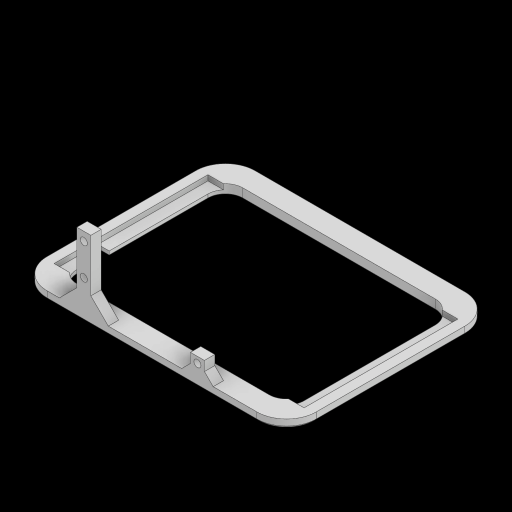
# Autodesk Inventor part: 220_Frame_Mainboard
Saved by Autodesk Inventor 2024 (Build 280153000, 153)
## iProperties
Created: 2023-07-20
Part Number: 220_Frame_Mainboard
Material: Generisch
Document SubType Name: Modeling
Designer: Philipp
Density: 1 g/cm^3
Appearance: Vorgabe
Author: Philipp
Autodesk Inventor part; units mm, degrees
ref_plane "YZ Plane" through (0, 0, 0) normal (1, 0, 0) x (0, 1, 0)
ref_plane "XZ Plane" through (0, 0, 0) normal (0, 1, 0) x (-1, 0, 0)
ref_plane "XY Plane" through (0, 0, 0) normal (0, 0, 1) x (1, 0, 0)
sketch "Skizze1" plane through (0, 0, 0) normal (0, 0, 1) x (1, 0, 0)
  line L0 (-77, 59.5) -> (77, 59.5)
  line L1 (77, 59.5) -> (77, -59.5)
  line L2 (77, -59.5) -> (-77, -59.5)
  line L3 (-77, -59.5) -> (-77, 59.5)
  line L4 (-77, 59.5) -> (77, -59.5) construction
  line L5 (77, 59.5) -> (-77, -59.5) construction
  point P0 (0, 0)
  dimension "d0" = 154
  dimension "d1" = 119
  constraints: 12 end point, 2 midpoint, 2 parallel, 1 horizontal, 1 perpendicular
  measures "d0" distance of L1.end L2.end
  measures "d1" distance of L0.end L1.end
extrude "Extrusion1" add sketch "Skizze1" along normal blind 5
fillet "Rundung1" radius 17 4 edges at (77, 59.5, 2.5) (77, -59.5, 2.5) (-77, -59.5, 2.5) (-77, 59.5, 2.5)
chamfer "Fasen1" distance 1.5 angle 45 8 edges at (-72.0208, 54.5208, 0) (-77, 0, 0) (-72.0208, -54.5208, 0) (0, -59.5, 0) (72.0208, -54.5208, 0) (77, 0, 0) (72.0208, 54.5208, 0) (0, 59.5, 0)
sketch "Skizze2" plane through (0, 0, 5) normal (0, 0, 1) x (1, 0, 0)
  line L0 (-55, 47.5) -> (55, 47.5)
  line L1 (65, 37.5) -> (65, -37.5)
  line L2 (55, -47.5) -> (-55, -47.5)
  line L3 (-65, -37.5) -> (-65, 37.5)
  line L4 (-65, 47.5) -> (65, -47.5) construction
  line L5 (65, 47.5) -> (-65, -47.5) construction
  arc A0 (-55, 47.5) -> (-65, 37.5) centre (-55, 37.5) ccw
  arc A1 (65, 37.5) -> (55, 47.5) centre (55, 37.5) ccw
  arc A2 (-65, -37.5) -> (-55, -47.5) centre (-55, -37.5) ccw
  arc A3 (55, -47.5) -> (65, -37.5) centre (55, -37.5) ccw
  line L6 (77, -42.5) -> (77, 42.5) projected
  line L7 (-77, 42.5) -> (-77, -42.5) projected
  line L8 (-60, -59.5) -> (60, -59.5) projected
  line L9 (60, 59.5) -> (-60, 59.5) projected
  point P0 (0, 0)
  dimension "d10" = 10
  dimension "d11" = 10
  dimension "d12" = 10
  dimension "d13" = 10
  dimension "d14" = 95
  dimension "d15" = 130
  dimension "d16" = 154
  dimension "d17" = 119
  constraints: 12 end point, 8 point on circle, 8 point on line, 8 tangent, 4 centre point, 2 midpoint, 2 parallel, 1 horizontal, 1 perpendicular
  measures "d10" radius of A0
  measures "d11" radius of A1
  measures "d12" radius of A2
  measures "d13" radius of A3
  measures "d14" distance between parallel lines of L2 L0
  measures "d15" distance between parallel lines of L3 L1
  measures "d16" distance between parallel lines of L6 L7
  measures "d17" distance between parallel lines of L8 L9
extrude "Extrusion2" cut sketch "Skizze2" against normal through all
sketch "Skizze3" plane through (0, 0, 5) normal (0, 0, 1) x (1, 0, 0)
  line L0 (-71.5, 44) -> (71.5, 44)
  line L1 (71.5, 44) -> (71.5, -44)
  line L2 (71.5, -44) -> (-71.5, -44)
  line L3 (-71.5, -44) -> (-71.5, 44)
  line L4 (-71.5, 44) -> (71.5, -44) construction
  line L5 (71.5, 44) -> (-71.5, -44) construction
  point P0 (0, 0)
  dimension "d20" = 143
  dimension "d21" = 88
  constraints: 12 end point, 2 midpoint, 2 parallel, 1 horizontal, 1 perpendicular
  measures "d20" distance of L1.end L2.end
  measures "d21" distance of L0.end L1.end
extrude "Extrusion3" cut sketch "Skizze3" against normal blind 3
sketch "Skizze5" plane through (0, 0, 5) normal (0, 0, 1) x (1, 0, 0)
  line L0 (-77, 42.5) -> (-77, -42.5) projected
  line L1 (-35, -59.5) -> (-43, -59.5)
  line L2 (-43, -59.5) -> (-43, -53.6)
  line L3 (-43, -53.6) -> (-35, -53.6)
  line L4 (-35, -53.6) -> (-35, -59.5)
  line L5 (-35, -59.5) -> (-43, -53.6) construction
  line L6 (-43, -59.5) -> (-35, -53.6) construction
  line L7 (-60, -59.5) -> (60, -59.5) projected
  line L8 (30, -59.5) -> (22, -59.5)
  line L9 (22, -59.5) -> (22, -53.6)
  line L10 (22, -53.6) -> (30, -53.6)
  line L11 (30, -53.6) -> (30, -59.5)
  line L12 (30, -59.5) -> (22, -53.6) construction
  line L13 (22, -59.5) -> (30, -53.6) construction
  point P0 (0, 0)
  point P1 (-39, -56.55)
  point P2 (26, -56.55)
  dimension "d29" = 38
  dimension "d30" = 5.9
  dimension "d31" = 8
  dimension "d37" = 103
  dimension "d38" = 8
  dimension "d39" = 5.9
  constraints: 24 end point, 4 midpoint, 4 parallel, 2 collinear, 2 horizontal, 2 perpendicular
  measures "d29" distance from line of L0 point (-39, -56.55)
  measures "d30" distance of L3.end L1.start
  measures "d31" distance of L2.end L3.end
  measures "d37" distance from line of L0 point (26, -56.55)
  measures "d38" distance of L8.start L8.end
  measures "d39" distance of L10.end L8.start
extrude "Extrusion5" add sketch "Skizze5" along normal blind 40 contours L1 L2 L3 L4
chamfer "Fasen2" distance 10 angle 45 2 edges at (-43, -56.55, 5) (-35, -56.55, 5)
sketch "Skizze6" plane through (0, 0, 5) normal (0, 0, 1) x (1, 0, 0)
  line L0 (22, -53.6) -> (30, -53.6) projected
  line L1 (30, -53.6) -> (30, -59.5) projected
  line L2 (30, -59.5) -> (22, -59.5) projected
  line L3 (22, -59.5) -> (22, -53.6) projected
  point P0 (0, 0)
extrude "Extrusion6" add sketch "Skizze6" along normal blind 10.5
chamfer "Fasen3" distance 5 angle 45 2 edges at (22, -56.55, 5) (30, -56.55, 5)
sketch "Skizze7" plane through (0, 0, 2) normal (0, 0, 1) x (1, 0, 0)
  line L0 (-65, -27) -> (-70, -27)
  line L1 (-70, -27) -> (-70, -19)
  line L2 (-70, -19) -> (-65, -19)
  line L3 (-65, -19) -> (-65, -27)
  line L4 (-65, -27) -> (-70, -19) construction
  line L5 (-70, -27) -> (-65, -19) construction
  line L6 (-62.5993, -44) -> (-71.5, -44) projected
  line L7 (-65, 37.5) -> (-65, -37.5) projected
  point P0 (0, 0)
  point P1 (-67.5, -23)
  dimension "d45" = 21
  dimension "d46" = 8
  dimension "d48" = 5
  constraints: 12 end point, 2 midpoint, 2 parallel, 1 collinear, 1 horizontal, 1 perpendicular
  measures "d45" distance from line of L6 point (-67.5, -23)
  measures "d46" distance of L2.end L0.start
  measures "d48" distance of L1.end L2.end
extrude "Extrusion7" cut sketch "Skizze7" against normal blind 3
sketch "Skizze8" plane through (22, -53.6, 15.5) normal (0, 1, 0) x (1, 0, 0)
  line L0 (-57, -29.5) -> (-65, -29.5) projected
  circle A0 centre (-61, -24.5) radius 2
  circle A1 centre (-61, -6.5) radius 2
  circle A2 centre (4, 3.5) radius 2
  line L1 (8, 0) -> (0, 0) projected
  line L2 (-61, -29.5) -> (-61, 10.5) construction
  line L3 (-77, 10.5) -> (33, 10.5) construction
  point P0 (-22, 15.5)
  point P1 (4, 0)
  dimension "d51" = 4
  dimension "d52" = 5
  dimension "d53" = 4
  dimension "d54" = 18
  dimension "d55" = 4
  dimension "d56" = 33
  dimension "d57" = 0
  constraints: 3 centre point, 3 point on line, 2 end point, 2 midpoint, 1 vertical
  measures "d51" diameter of A0
  measures "d52" distance from line of L0 A0.centre
  measures "d53" diameter of A1
  measures "d54" distance of A0.centre A1.centre
  measures "d55" diameter of A2
  measures "d56" distance from line of L0 A2.centre
  measures "d57" horizontal distance of point (4, 0) A2.centre
extrude "Extrusion8" cut sketch "Skizze8" against normal through all
